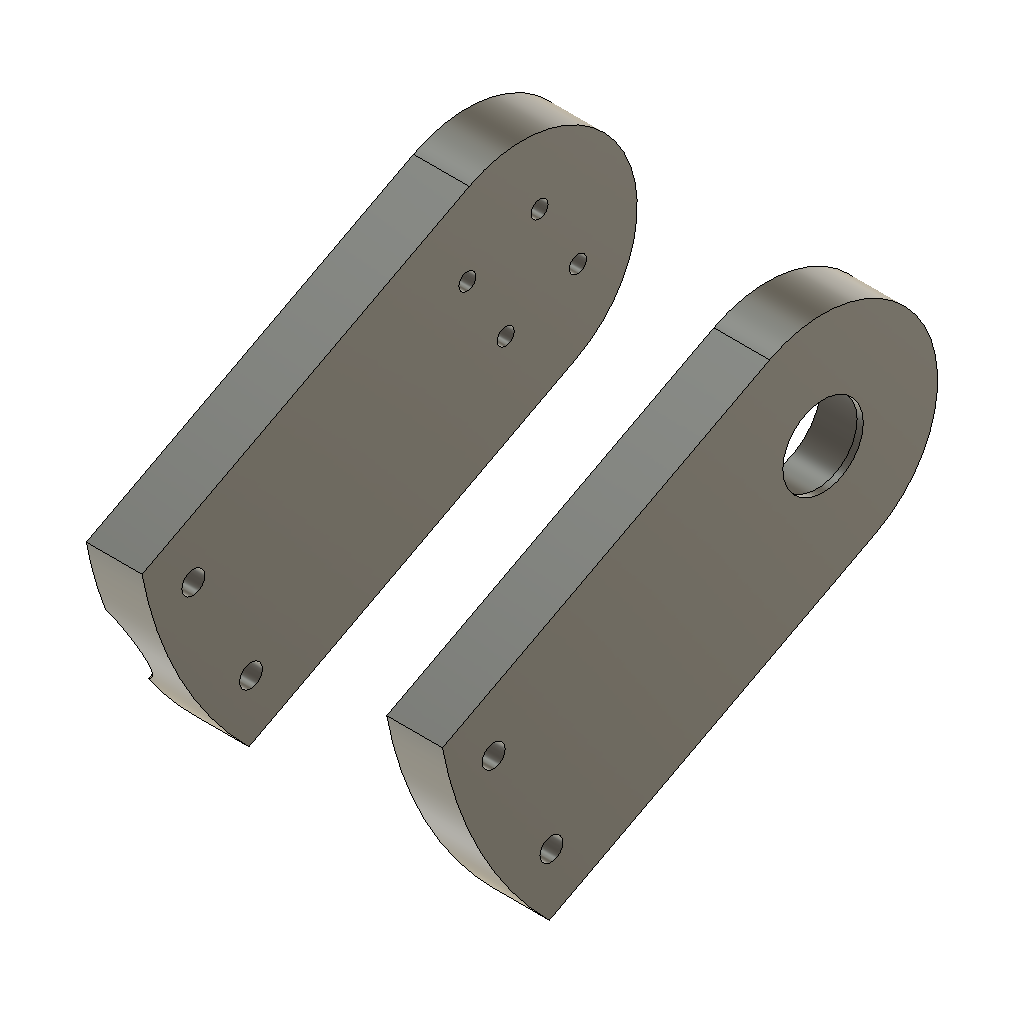
weapon-arms (Autodesk Fusion 360 design; units mm, degrees)
Autodesk Fusion 360 part; units mm, degrees
sketch "arm-weapon" plane through (0, 0, 0) normal (1, 0, 0) x (0, 1, 0)
  circle A0 centre (0, 0) radius 62.5
  line L0 (-61.4416, -11.4536) -> (-8.6216, 16.3682)
  line L1 (-44.1983, -44.19) -> (8.6216, -16.3682)
  arc A1 (8.6216, -16.3682) -> (-8.6216, 16.3682) centre (0, 0) ccw
  line L2 (-8.6216, 16.3682) -> (0, 0)
  circle A2 centre (0, 0) radius 15
  line L3 (-7.9982, -12.6897) -> (-14.9887, 0.5818)
  line L4 (-14.9887, 0.5818) -> (-28.2602, -6.4087)
  line L5 (-28.2602, -6.4087) -> (-21.2697, -19.6802)
  line L6 (-21.2697, -19.6802) -> (-7.9982, -12.6897)
  line L7 (-11.4935, -6.0539) -> (0, 0)
  line L8 (-61.4416, -11.4536) -> (-44.1983, -44.19)
  circle A3 centre (-53.1715, -16.7046) radius 1.85
  circle A4 centre (-43.8508, -34.3999) radius 1.85
  line L9 (-34.5302, -52.0953) -> (-62.4921, 0.9908)
  point P0 (-52.8199, -27.8218)
  point P1 (-48.5112, -25.5523)
  dimension "d1" = 125
  dimension "d2" = 30
  dimension "d3" = 3.5
  dimension "d9" = 15
  dimension "d11" = 15
  dimension "d12" = 3.7
  dimension "d13" = 3.7
  dimension "d28" = 60
  dimension "d29" = 10
  dimension "d30" = 10
  constraint coincident A0.centre A1.centre
  constraint coincident A0 L0.start
  constraint coincident A0 L1.start
  constraint parallel L0 L1
  constraint coincident L1.end A1.start
  constraint collinear L0.end L1.end A0.centre
  constraint perpendicular L0 L2
  constraint concentric A1 A2
  constraint coincident A2 L3.start
  constraint coincident A2 L3.end
  constraint parallel L3 L5
  constraint parallel L4 L6
  constraint parallel L0 L4
  constraint midpoint L3 L7.start
  constraint parallel L4 L7
  constraint coincident A0 L9.start
  constraint coincident A0 L9.end
  constraint coincident A4.centre L9
  constraint coincident A3.centre L9
  constraint midpoint L9 P1
  measures "d1" diameter of A0
  measures "d2" diameter of A2
  measures "d3" distance of A1 A2
  measures "d9" distance of L3.start L5.end
  measures "d11" distance of L4.end L5.end
  measures "d12" diameter of A3
  measures "d13" diameter of A4
  measures "d28" distance of L9.start L9.end
  measures "d29" distance of A3.centre P1
  measures "d30" distance of A4.centre P1
extrude "Extrude1" add sketch "arm-weapon" along normal blind 2.5 contours A0 L8 | L0 L1 L8 A3 A4 L9 | L0 L1 A1 A3 A4 L9 | L2 A2 L3 L7 | L2 A2 L3 L7 | A2 L3 | A2 L4 L5 L6 makes body 1
extrude "Extrude2" add sketch "arm-weapon" against normal blind 6.5 contours A0 L8 | L0 L1 L8 A3 A4 L9 | L0 L1 A1 A3 A4 L9 bodies 1
sketch "Sketch2" plane through (0, 0, 0) normal (1, 0, 0) x (0, 1, 0)
  circle A0 centre (0, 0) radius 62.5
  circle A1 centre (0, 0) radius 18.5
  line L0 (-8.6216, 16.3682) -> (-61.4395, -11.4647)
  line L1 (-44.1904, -44.198) -> (8.6246, -16.3666)
  line L2 (-61.4395, -11.4647) -> (-44.1904, -44.198)
  circle A2 centre (-53.1715, -16.7046) radius 1.85
  circle A3 centre (-43.8508, -34.3999) radius 1.85
  circle A4 centre (0, 0) radius 8.75
  circle A5 centre (0, 0) radius 6.5
  line L3 (-62.4921, 0.9908) -> (-34.5302, -52.0953)
  line L4 (-61.4416, -11.4536) -> (-44.1983, -44.19)
  point P0 (-8.6216, 16.3682)
  point P1 (-52.8149, -27.8313)
  point P2 (-48.5112, -25.5523)
  dimension "d16" = 3.7
  dimension "d17" = 3.7
  dimension "d20" = 17.5
  dimension "d21" = 2.25
  dimension "d38" = 125
  dimension "d39" = 60
  dimension "d40" = 10
  dimension "d41" = 10
  constraint coincident A0.centre A1.centre
  constraint concentric A0 A1
  constraint coincident A1 P0
  constraint coincident P0 L0.start
  constraint coincident A0 L0.end
  constraint tangent A1 L0
  constraint coincident A0 L1.start
  constraint coincident A1 L1.end
  constraint tangent A1 L1
  constraint parallel L0 L1
  constraint midpoint L2 P1
  constraint concentric A1 A4
  constraint concentric A1 A5
  constraint coincident A0 L3.start
  constraint coincident A0 L3.end
  constraint parallel L3 L4
  constraint coincident A2.centre L3
  constraint coincident A3.centre L3
  measures "d16" diameter of A2
  measures "d17" diameter of A3
  measures "d20" diameter of A4
  measures "d21" distance of A4 A5
  measures "d38" diameter of A0
  measures "d39" distance of L3.start L3.end
  measures "d40" distance of A2.centre P2
  measures "d41" distance of A3.centre P2
extrude "Extrude3" add sketch "Sketch2" along normal blind 1 separate body contours A1 | L0 L1 L2 A2 A3 L3 L4 | A1 L0 L1 A2 A3 L3 | A0 L2 L4 | A0 L2 L4 | L0 L2 L4 | A4 makes body 2
extrude "Extrude4" add sketch "Sketch2" against normal blind 8 contours A1 | L0 L1 L2 A2 A3 L3 L4 | A1 L0 L1 A2 A3 L3 | A0 L2 L4 | A0 L2 L4 | L0 L2 L4 bodies 2
move_body "Move1" bodies 2 to x (1, 0, 0) y (0, 1, 0) z (0, 0, 1) at (50, 0, 0)
fillet "Fillet1" radius 3 2 edges at (-3.25, -14.9887, 0.5818) (-3.25, -7.9982, -12.6897) on bodies 1
sketch "Sketch3" plane through (0, -24.765, -13.0444) normal (0, 0.884767, 0.466033) x (-1, 0, 0)
  line L0 (0, 7.5) -> (0, -7.5)
  line L1 (0, -7.5) -> (6.5, -7.5)
  line L2 (6.5, -7.5) -> (6.5, 7.5)
  line L3 (6.5, 7.5) -> (0, 7.5)
  arc A0 (6.5, 7.5) -> (6.5, -7.5) centre (13.1144, 0) ccw
  dimension "d33" = 10
  constraint coincident L1.end L2.start
  constraint coincident L2.end L3.start
  measures "d33" radius of A0
extrude "Extrude5" cut sketch "Sketch3" along normal up to surface contours L2 A0 end surface at (-0.5, -45.9329, -42.3841) on bodies 1 bodies 1
fillet "Fillet2" radius 5 2 edges at (0, -24.765, -13.0444) (-3.1144, -24.765, -13.0444) on bodies 1
sketch "Sketch4" plane through (2.5, 0, 0) normal (1, 0, 0) x (0, 1, 0)
  circle A0 centre (-43.8508, -34.3999) radius 1.85
  circle A1 centre (-53.1715, -16.7046) radius 1.85
  arc A2 (-61.4416, -11.4536) -> (-44.1983, -44.19) centre (0, 0) ccw
  line L0 (-44.1983, -44.19) -> (8.6216, -16.3682)
  arc A3 (8.6216, -16.3682) -> (-8.6216, 16.3682) centre (0, 0) ccw
  line L1 (-8.6216, 16.3682) -> (-61.4416, -11.4536)
  circle A4 centre (-3.8036, 8.1568) radius 2.5
  circle A5 centre (8.1568, 3.8036) radius 2.5
  circle A6 centre (0, 0) radius 12.3006
  circle A7 centre (-8.1568, -3.8036) radius 2.5
  circle A8 centre (3.8036, -8.1568) radius 2.5
  circle A9 centre (0, 0) radius 5.1688
  circle A10 centre (-8.9271, 3.2492) radius 1.375
  circle A11 centre (2.7362, 7.5175) radius 1.375
  circle A12 centre (-2.7362, -7.5175) radius 1.375
  circle A13 centre (8.9271, -3.2492) radius 1.375
  dimension "d42" = 2.75
  dimension "d43" = 2.75
  dimension "d44" = 2.75
  dimension "d45" = 2.75
  measures "d42" diameter of A10
  measures "d43" diameter of A11
  measures "d44" diameter of A12
  measures "d45" diameter of A13
extrude "Extrude6" cut sketch "Sketch4" against normal blind 19 contours A10 | A11 | A12 | A13 bodies 1
sketch "Sketch5" plane through (-6.5, 0, 0) normal (-1, 0, 0) x (0, -1, 0)
  line L0 (16.4307, -0.1777) -> (32.6841, -8.7389)
  line L1 (32.6841, -8.7389) -> (58.3936, -22.2808)
  arc A0 (58.3936, -22.2808) -> (61.4416, -11.4536) centre (0, 0) ccw
  line L2 (61.4416, -11.4536) -> (8.6216, 16.3682)
  arc A1 (8.6216, 16.3682) -> (-8.6216, -16.3682) centre (0, 0) ccw
  line L3 (-8.6216, -16.3682) -> (44.1983, -44.19)
  arc A2 (44.1983, -44.19) -> (51.4031, -35.5523) centre (0, 0) ccw
  line L4 (51.4031, -35.5523) -> (25.6936, -22.0104)
  line L5 (25.6936, -22.0104) -> (9.4402, -13.4492)
  arc A3 (9.4402, -13.4492) -> (6.7018, -13.4196) centre (8.0421, -16.1035) ccw
  arc A4 (14.8573, 2.0638) -> (6.7018, -13.4196) centre (0, 0) ccw
  arc A5 (14.8573, 2.0638) -> (16.4307, -0.1777) centre (17.8288, 2.4766) ccw
  circle A6 centre (43.8508, -34.3999) radius 1.85
  circle A7 centre (53.1715, -16.7046) radius 1.85
  circle A8 centre (53.1715, -16.7046) radius 4.5
  circle A9 centre (43.8508, -34.3999) radius 4.5
  dimension "d49" = 9
  dimension "d50" = 9
  constraint concentric A7 A8
  constraint concentric A6 A9
  measures "d49" diameter of A8
  measures "d50" diameter of A9
extrude "Extrude7" cut sketch "Sketch5" against normal blind 6 contours L1 A8 | L1 A8 | L4 A9 | L4 A9 bodies 1
sketch "Sketch6" plane through (42, 0, 0) normal (-1, 0, 0) x (0, -1, 0)
  circle A0 centre (53.1715, -16.7046) radius 1.85
  circle A1 centre (0, 0) radius 8.75
  circle A2 centre (43.8508, -34.3999) radius 1.85
  line L0 (-8.6246, -16.3666) -> (44.1904, -44.198)
  arc A3 (44.1904, -44.198) -> (61.4395, -11.4647) centre (0, 0) ccw
  line L1 (61.4395, -11.4647) -> (8.6263, 16.3657)
  arc A4 (8.6263, 16.3657) -> (-8.6246, -16.3666) centre (0, 0) ccw
  circle A5 centre (53.1715, -16.7046) radius 4.5
  circle A6 centre (43.8508, -34.3999) radius 4.5
  dimension "d53" = 9
  dimension "d54" = 9
  constraint concentric A0 A5
  constraint concentric A2 A6
  measures "d53" diameter of A5
  measures "d54" diameter of A6
extrude "Extrude8" cut sketch "Sketch6" against normal blind 6 contours A5 | A6 bodies 2
equation "d42 = d44"
equation "d44 = d43"
equation "d45 = d43"
